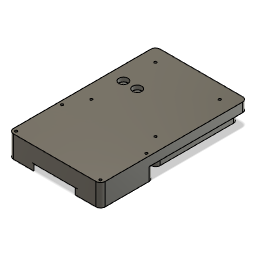
Base A v9 fix v3 (Autodesk Fusion 360 design; units mm, degrees)
Autodesk Fusion 360 part; units mm, degrees
sketch "スケッチ1" plane through (0, 0, 0) normal (0, 1, 0) x (1, 0, 0)
  line L0 (-100, 0) -> (100, 0) construction
  line L1 (0, 100) -> (0, -150) construction
  line L2 (-40, 40) -> (40, 40)
  line L3 (40, 40) -> (40, -40)
  line L4 (40, -40) -> (-40, -40)
  line L5 (-40, -40) -> (-40, 40)
  line L6 (-40, 9.5) -> (-12, 9.5)
  line L7 (-12, 9.5) -> (-12, -9.5)
  line L8 (-12, -9.5) -> (-40, -9.5)
  line L9 (-40, -9.5) -> (-40, 9.5)
  circle A0 centre (-35, 0) radius 2.5
  circle A1 centre (-20, 0) radius 2.5
  circle A2 centre (0, 0) radius 35 construction
  circle A3 centre (0, 0) radius 40 construction
  circle A4 centre (-35, 35) radius 1.25
  circle A5 centre (35, 35) radius 1.25
  circle A6 centre (-35, -35) radius 1.25
  circle A7 centre (35, -35) radius 1.25
  circle A8 centre (-35, 0) radius 5
  circle A9 centre (-20, 0) radius 5
  line L10 (-50, -52) -> (50, -52)
  line L11 (50, -52) -> (50, 50)
  line L12 (50, 50) -> (-50, 50)
  line L13 (-50, 50) -> (-50, -52)
  line L14 (50, -52) -> (-50, -52)
  line L15 (-50, -52) -> (-50, -110)
  line L16 (-50, -110) -> (50, -110)
  line L17 (50, -110) -> (50, -52)
  line L18 (27.5, -110) -> (-27.5, -110)
  line L19 (-27.5, -110) -> (-27.5, -55)
  line L20 (-27.5, -55) -> (27.5, -55)
  line L21 (27.5, -55) -> (27.5, -110)
  line L22 (48, -54) -> (48, -108)
  line L23 (48, -108) -> (-48, -108)
  line L24 (-48, -108) -> (-48, -54)
  line L25 (43, -43) -> (-43, -43)
  line L26 (-43, -43) -> (-43, 43)
  line L27 (-43, 43) -> (43, 43)
  line L28 (43, 43) -> (43, -43)
  line L29 (-40, -9.5) -> (-43, -9.5)
  line L30 (-40, 9.5) -> (-43, 9.5)
  line L31 (45, -45) -> (-45, -45)
  line L32 (-45, -45) -> (-45, 45)
  line L33 (-45, 45) -> (45, 45)
  line L34 (45, 45) -> (45, -45)
  line L35 (48, -54) -> (-48, -54)
  line L36 (10, -55) -> (10, -40)
  line L37 (-10, -55) -> (-10, -40)
  circle A10 centre (46, -106) radius 1.25
  circle A11 centre (46, -56) radius 1.25
  circle A12 centre (-46, -106) radius 1.25
  circle A13 centre (-46, -56) radius 1.25
  circle A14 centre (46, -106) radius 4
  circle A15 centre (46, -56) radius 4
  circle A16 centre (-46, -106) radius 4
  circle A17 centre (-46, -56) radius 4
  line L38 (36.7, -77) -> (-39.3, -77) construction
  line L39 (-39.3, -77) -> (-39.3, -61) construction
  line L40 (-39.3, -61) -> (36.7, -61) construction
  line L41 (36.7, -61) -> (36.7, -77) construction
  circle A18 centre (36.7, -61) radius 0.9
  circle A19 centre (36.7, -61) radius 4
  circle A20 centre (36.7, -77) radius 0.9
  circle A21 centre (36.7, -77) radius 4
  circle A22 centre (-39.3, -61) radius 0.9
  circle A23 centre (-39.3, -61) radius 4
  circle A24 centre (-39.3, -77) radius 0.9
  circle A25 centre (-39.3, -77) radius 4
  line L42 (27.5, -100) -> (-27.5, -100)
  line L43 (-42.127, -107) -> (42.127, -107)
  line L44 (-47, -102.127) -> (-47, -59.873)
  line L45 (47, -102.127) -> (47, -59.873)
  line L46 (-42.127, -55) -> (42.127, -55)
  arc A26 (-27.5, -105) -> (-22.5, -110) centre (-22.5, -105) ccw
  arc A27 (-22.5, -55) -> (-27.5, -60) centre (-22.5, -60) ccw
  arc A28 (27.5, -60) -> (22.5, -55) centre (22.5, -60) ccw
  arc A29 (22.5, -110) -> (27.5, -105) centre (22.5, -105) ccw
  line L47 (-35.3, -77) -> (-35.3, -61)
  line L48 (-43.3, -77) -> (-43.3, -61)
  line L49 (32.7, -77) -> (32.7, -61)
  line L50 (40.7, -77) -> (40.7, -61)
  line L51 (-43, -14.5) -> (43, -14.5)
  line L52 (43, -14.5) -> (43, -9.5)
  line L53 (43, -9.5) -> (-43, -9.5)
  line L54 (-43, -9.5) -> (-43, -14.5)
  line L55 (-43, 9.5) -> (43, 9.5)
  line L56 (43, 9.5) -> (43, 14.5)
  line L57 (43, 14.5) -> (-43, 14.5)
  line L58 (-43, 14.5) -> (-43, 9.5)
  line L59 (-2.5, -43) -> (2.5, -43)
  line L60 (2.5, -43) -> (2.5, 43)
  line L61 (2.5, 43) -> (-2.5, 43)
  line L62 (-2.5, 43) -> (-2.5, -43)
  dimension "d1" = 40
  dimension "d2" = 40
  dimension "d3" = 40
  dimension "d4" = 40
  dimension "d5" = 5
  dimension "d6" = 5
  dimension "d7" = 15
  dimension "d8" = 5
  dimension "d9" = 28
  dimension "d10" = 9.5
  dimension "d11" = 9.5
  dimension "d12" = 70
  dimension "d13" = 80
  dimension "d14" = 2.5
  dimension "d15" = 2.5
  dimension "d16" = 2.5
  dimension "d17" = 2.5
  dimension "d18" = 5
  dimension "d19" = 5
  dimension "d20" = 5
  dimension "d21" = 5
  dimension "d22" = 5
  dimension "d23" = 5
  dimension "d24" = 5
  dimension "d25" = 5
  dimension "d26" = 10
  dimension "d27" = 10
  dimension "d56" = 52
  dimension "d57" = 50
  dimension "d58" = 50
  dimension "d59" = 50
  dimension "d60" = 58
  dimension "d61" = 100
  dimension "d62" = 55
  dimension "d63" = 55
  dimension "d64" = 27.5
  dimension "d65" = 2
  dimension "d66" = 2
  dimension "d67" = 2
  dimension "d68" = 7
  dimension "d69" = 7
  dimension "d70" = 9
  dimension "d71" = 7
  dimension "d72" = 2
  dimension "d73" = 2
  dimension "d74" = 2
  dimension "d75" = 2
  dimension "d76" = 2
  dimension "d77" = 2.5
  dimension "d78" = 4
  dimension "d79" = 4
  dimension "d80" = 2.5
  dimension "d81" = 4
  dimension "d82" = 4
  dimension "d83" = 2.5
  dimension "d84" = 4
  dimension "d85" = 4
  dimension "d86" = 2.5
  dimension "d87" = 4
  dimension "d88" = 4
  dimension "d89" = 8
  dimension "d90" = 8
  dimension "d91" = 8
  dimension "d92" = 8
  dimension "d93" = 27.5
  dimension "d94" = 76
  dimension "d95" = 16
  dimension "d96" = 1.8
  dimension "d97" = 8
  dimension "d98" = 1.8
  dimension "d99" = 8
  dimension "d100" = 1.8
  dimension "d101" = 8
  dimension "d102" = 1.8
  dimension "d103" = 8
  dimension "d104" = 36.7
  dimension "d107" = 39.3
  dimension "d108" = 6
  dimension "d131" = 10
  dimension "d138" = 1
  dimension "d139" = 1
  dimension "d140" = 1
  dimension "d141" = 1
  dimension "d144" = 40
  dimension "d145" = 40
  dimension "d146" = 5
  dimension "d147" = 5
  dimension "d148" = 5
  dimension "d149" = 5
  dimension "d150" = 5
  dimension "d151" = 5
  dimension "d152" = 5
  dimension "d153" = 5
  dimension "d155" = 5
  dimension "d156" = 25.5
  dimension "d157" = 25.5
  dimension "d158" = 5
  dimension "d159" = 2.5
  dimension "d160" = 2.5
  constraint horizontal L0
  constraint perpendicular L0 L1
  constraint horizontal L2
  constraint vertical L3
  constraint horizontal L4
  constraint vertical L5
  constraint horizontal L6
  constraint vertical L7
  constraint horizontal L8
  constraint vertical L9
  constraint coincident L5 L6.start
  constraint coincident L0 A0.centre
  constraint coincident L0 A1.centre
  constraint coincident A2.centre A3.centre
  constraint concentric A2 A3
  constraint concentric A0 A8
  constraint concentric A1 A9
  constraint horizontal L10
  constraint vertical L11
  constraint horizontal L12
  constraint vertical L13
  constraint horizontal L14
  constraint vertical L15
  constraint horizontal L16
  constraint vertical L17
  constraint horizontal L18
  constraint vertical L19
  constraint horizontal L20
  constraint vertical L21
  constraint coincident L16 L18.start
  constraint perpendicular L16 L22
  constraint perpendicular L22 L23
  constraint perpendicular L10 L24
  constraint horizontal L25
  constraint vertical L26
  constraint horizontal L27
  constraint vertical L28
  constraint coincident L26 L29.end
  constraint perpendicular L26 L29
  constraint coincident L26 L30.end
  constraint perpendicular L26 L30
  constraint horizontal L31
  constraint vertical L32
  constraint horizontal L33
  constraint vertical L34
  constraint coincident L22 L35.start
  constraint coincident L24 L35.end
  constraint perpendicular L24 L35
  constraint coincident L4 L36.end
  constraint perpendicular L4 L36
  constraint coincident L4 L37.end
  constraint perpendicular L4 L37
  constraint concentric A10 A14
  constraint concentric A11 A15
  constraint concentric A12 A16
  constraint concentric A13 A17
  constraint horizontal L38
  constraint vertical L39
  constraint horizontal L40
  constraint vertical L41
  constraint coincident L40.end L41.start
  constraint concentric A18 A19
  constraint coincident L38.start L41.end
  constraint concentric A20 A21
  constraint coincident L39.end L40.start
  constraint concentric A22 A23
  constraint coincident L38.end L39.start
  constraint concentric A24 A25
  constraint perpendicular L19 L42
  constraint coincident L19 L42.end
  constraint coincident L21 L42.start
  constraint coincident A16 L43.start
  constraint coincident A14 L43.end
  constraint horizontal L43
  constraint coincident A16 L44.start
  constraint coincident A17 L44.end
  constraint vertical L44
  constraint coincident A14 L45.start
  constraint coincident A15 L45.end
  constraint parallel L22 L45
  constraint coincident A17 L46.start
  constraint coincident A15 L46.end
  constraint perpendicular L36 L46
  constraint coincident L37.start L46
  constraint coincident L36.start L46
  constraint coincident L18 A26.end
  constraint tangent L16 A26
  constraint coincident L20 A27.start
  constraint coincident L20 A28.end
  constraint coincident L18 A29.start
  constraint tangent L20 A27
  constraint tangent L20 A28
  constraint tangent L21 A29
  constraint coincident L38 L47.start
  constraint coincident A25 L47.start
  constraint coincident L40 L47.end
  constraint coincident A23 L47.end
  constraint coincident A25 L48.start
  constraint coincident A23 L48.end
  constraint tangent A23 L48
  constraint perpendicular L40 L48
  constraint coincident L38 L49.start
  constraint coincident A21 L49.start
  constraint coincident A19 L49.end
  constraint coincident L40 L49.end
  constraint coincident A21 L50.start
  constraint coincident A19 L50.end
  constraint tangent A19 L50
  constraint perpendicular L40 L50
  constraint horizontal L51
  constraint vertical L52
  constraint horizontal L53
  constraint vertical L54
  constraint coincident L28 L52.end
  constraint coincident L26 L51.start
  constraint horizontal L55
  constraint vertical L56
  constraint horizontal L57
  constraint vertical L58
  constraint coincident L28 L56.end
  constraint horizontal L59
  constraint vertical L60
  constraint horizontal L61
  constraint vertical L62
  constraint coincident L27 L60.end
  constraint coincident L25 L59.start
  measures "d1" distance of L0 L2
  measures "d2" distance of L0 L4
  measures "d3" distance of L1 L5
  measures "d4" distance of L1 L3
  measures "d5" diameter of A0
  measures "d6" diameter of A1
  measures "d7" distance of A0.centre A1.centre
  measures "d8" distance of L5 A0.centre
  measures "d9" distance of L7 L9
  measures "d10" distance of L0 L6
  measures "d11" distance of L0 L8
  measures "d12" diameter of A2
  measures "d13" diameter of A3
  measures "d14" diameter of A4
  measures "d15" diameter of A5
  measures "d16" diameter of A6
  measures "d17" diameter of A7
  measures "d18" distance of L2 A4.centre
  measures "d19" distance of L5 A4.centre
  measures "d20" distance of L2 A5.centre
  measures "d21" distance of L3 A5.centre
  measures "d22" distance of L4 A6.centre
  measures "d23" distance of L5 A6.centre
  measures "d24" distance of L3 A7.centre
  measures "d25" distance of L4 A7.centre
  measures "d26" diameter of A8
  measures "d27" diameter of A9
  measures "d56" distance of L0 L10
  measures "d57" distance of L0 L12
  measures "d58" distance of L1 L13
  measures "d59" distance of L1 L11
  measures "d60" distance of L14 L16
  measures "d61" distance of L15 L17
  measures "d62" distance of L19 L21
  measures "d63" distance of L18 L20
  measures "d64" distance of L1 L21
  measures "d65" distance of L17 L22
  measures "d66" distance of L16 L23
  measures "d67" distance of L15 L24
  measures "d68" distance of L11 L28
  measures "d69" distance of L12 L27
  measures "d70" distance of L14 L25
  measures "d71" distance of L13 L26
  measures "d72" distance of L27 L33
  measures "d73" distance of L28 L34
  measures "d74" distance of L25 L31
  measures "d75" distance of L26 L32
  measures "d76" distance of L10 L35
  measures "d77" diameter of A10
  measures "d78" distance of L16 A10.centre
  measures "d79" distance of L17 A10.centre
  measures "d80" diameter of A11
  measures "d81" distance of L17 A11.centre
  measures "d82" distance of L14 A11.centre
  measures "d83" diameter of A12
  measures "d84" distance of L15 A12.centre
  measures "d85" distance of L16 A12.centre
  measures "d86" diameter of A13
  measures "d87" distance of L15 A13.centre
  measures "d88" distance of L10 A13.centre
  measures "d89" diameter of A14
  measures "d90" diameter of A15
  measures "d91" diameter of A16
  measures "d92" diameter of A17
  measures "d93" distance of L1 L19
  measures "d94" distance of L39 L41
  measures "d95" distance of L38 L40
  measures "d96" diameter of A18
  measures "d97" diameter of A19
  measures "d98" diameter of A20
  measures "d99" diameter of A21
  measures "d100" diameter of A22
  measures "d101" diameter of A23
  measures "d102" diameter of A24
  measures "d103" diameter of A25
  measures "d104" distance of L1 L41
  measures "d107" distance of L1 L39
  measures "d108" distance of L20 L40
  measures "d131" distance of L16 L42
  measures "d138" distance of L22 L45
  measures "d139" distance of L23 L43
  measures "d140" distance of L24 L44
  measures "d141" distance of L35 L46
  measures "d144" distance of L11 L36
  measures "d145" distance of L13 L37
  measures "d146" distance of L16 A26.centre
  measures "d147" distance of L19 A26.centre
  measures "d148" distance of L16 A29.centre
  measures "d149" distance of L21 A29.centre
  measures "d150" distance of L20 A28.centre
  measures "d151" distance of L21 A28.centre
  measures "d152" distance of L20 A27.centre
  measures "d153" distance of L19 A27.centre
  measures "d155" distance of L55 L57
  measures "d156" distance of L2 L57
  measures "d157" distance of L4 L51
  measures "d158" distance of L51 L53
  measures "d159" distance of L1 L62
  measures "d160" distance of L1 L60
extrude "押し出し1" add sketch "スケッチ1" against normal blind 2 contours L2 L5 L26 L27 L57 L62 | L2 L5 L57 L62 | L2 L27 L60 L61 L62 | L2 L57 L60 L62 | L5 L6 L55 L57 L62 | L5 L26 L30 L55 L57 L58 | L2 L3 L27 L28 L57 L60 | L2 L3 L57 L60 | L55 L57 L60 L62 | L3 L55 L57 L60 | L7 L53 L55 L62 | L53 L55 L60 L62 | L3 L28 L55 L56 L57 | L3 L53 L55 L60 | L5 L8 L51 L53 L62 | L51 L53 L60 L62 | L5 L26 L29 L51 L53 L54 | L3 L28 L53 L55 | L3 L51 L53 L60 | L4 L5 L51 L62 | L4 L51 L60 L62 | L4 L5 L25 L26 L37 L51 | L3 L28 L51 L52 L53 | L3 L4 L51 L60 | L4 L25 L37 L62 | L4 L25 L59 L60 L62 | L3 L4 L25 L28 L36 L51 | L4 L25 L36 L60 | L25 L31 L36 L37 L59 | L10 L14 L31 L36 L37 | L10 L14 L35 L36 L37 | L20 L35 L37 A17 L46 | L20 L35 L36 L37 L46 | L20 L35 L36 A15 L46 | L19 L20 L21 L42 L46 A27 A28 | L19 A16 A17 L43 L44 L46 | L24 A16 A17 L44 | L19 L20 L46 A27 | L22 A14 A15 L45 | L21 A14 A15 L43 L45 L46 | L20 L21 L46 A28 | L19 L23 A16 L43 | L21 L23 A14 L43 | A18 | A19 A21 L49 L50 | A20 | A22 | A23 A25 L47 L48 | A24 makes body 1 at (18.9872, 0, 3.1667) makes body 2 at (37.5293, -1.3333, 76.6504) makes body 3 at (-38.532, -1.3333, 60.5307) makes body 4 at (37.468, -1.3333, 60.5307) makes body 5 at (-38.4707, -1.3333, 76.6504)
extrude "押し出し2" add sketch "スケッチ1" against normal blind 9 contours L5 L6 L7 L8 L9 L53 L55 | L5 L9 L26 L29 L30 L53 L55 bodies 1
extrude "押し出し8" add sketch "スケッチ1" against normal blind 16 contours A19 | A19 A21 L49 L50 | A21 | A23 | A23 A25 L47 L48 | A25 bodies 1 3 2 5 4
extrude "押し出し11" add sketch "スケッチ1" against normal blind 10 contours L10 L11 L12 L13 L14 L31 L32 L33 L34 L36 L37 bodies 1
extrude "押し出し12" add sketch "スケッチ1" against normal blind 18 contours L25 L26 L27 L28 L31 L32 L33 L34 L36 L37 L52 L54 L56 L58 L61 bodies 1
extrude "押し出し3" add sketch "スケッチ1" against normal blind 2 from surface at -7 contours A8 | A9 bodies 1
fillet "フィレット1" radius 2.5 2 edges at (-39.6616, -7, -1.8081) (-24.6616, -7, -1.8081) on bodies 1
extrude "押し出し9" add sketch "スケッチ1" against normal blind 10 separate body contours L10 L11 L12 L13 L14 L31 L32 L33 L34 L36 L37 makes body 6
extrude "押し出し10" add sketch "スケッチ1" against normal blind 20 contours L25 L26 L27 L28 L31 L32 L33 L34 L36 L37 L52 L54 L56 L58 L61 bodies 1 6
fillet "フィレット2" radius 5 2 edges at (-50, -5, -50) (50, -5, -50) on bodies 1
fillet "フィレット3" radius 5 4 edges at (-45, -15, -45) (45, -15, -45) (45, -15, 45) (-45, -15, 45) on bodies 1
fillet "フィレット4" radius 3 4 edges at (-43, -11, -43) (43, -11, -43) (-43, -11, 43) (43, -11, 43) on bodies 1
extrude "押し出し13" add sketch "スケッチ1" against normal blind 24 contours L10 L14 L35 L37 A17 | L10 L14 L35 L36 A15 | L10 L14 L15 A17 | L24 L35 A17 | L10 L14 L17 A15 | L22 L35 A15 | L24 L35 A17 | L15 L24 A16 A17 | L17 L22 A14 A15 | L22 L35 A15 | L15 L16 A16 | L23 L24 A16 | L22 L23 A14 | L16 L17 A14 | L23 L24 A16 | L16 L19 L23 A16 | L22 L23 A14 | L16 L21 L23 A14 | L16 L18 L19 L23 A26 | L16 L18 L21 L23 A29 bodies 1
extrude "押し出し14" add sketch "スケッチ1" against normal blind 17.2 contours L16 L18 L19 L23 A26 | L19 L21 L42 L43 A26 A29 | L16 L18 L21 L23 A29 | L16 L18 L23 A26 A29 | L19 L23 L43 A26 | L19 L43 A26 | L21 L23 L43 A29 | L21 L43 A29 | L23 L43 A26 A29 bodies 1
fillet "フィレット6" radius 5 4 edges at (-50, -12, 110) (-50, -17, 52) (50, -17, 52) (50, -12, 110) on bodies 1
extrude "押し出し16" add sketch "スケッチ1" against normal blind 7 contours L5 L6 L55 L57 L62 | L5 L26 L30 L55 L57 L58 | L55 L57 L60 L62 | L3 L55 L57 L60 | L3 L28 L55 L56 L57 | L5 L8 L51 L53 L62 | L51 L53 L60 L62 | L5 L26 L29 L51 L53 L54 | L3 L51 L53 L60 | L3 L28 L51 L52 L53 bodies 1
extrude "押し出し17" add sketch "スケッチ1" against normal blind 5 contours L2 L27 L60 L61 L62 | L2 L57 L60 L62 | L53 L55 L60 L62 | L4 L51 L60 L62 | L4 L25 L59 L60 L62 bodies 1
extrude "押し出し18" add sketch "スケッチ1" against normal blind 5 contours L25 L31 L36 L37 L59 | L10 L14 L31 L36 L37 | L10 L14 L35 L36 L37 bodies 1
extrude "押し出し15" [suppressed]
